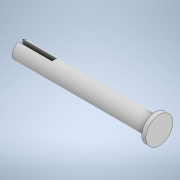
# Autodesk Inventor part: handle insert
Saved by Autodesk Inventor 2020.4 (Build 244396000, 396)
## iProperties
Created: 2023-07-18
Part Number: handle insert
Material: Generic
Document SubType Name: Modeling
Designer: Paul
Density: 1 g/cm^3
Appearance: Default
Author: Paul
Autodesk Inventor part; units mm, degrees
ref_plane "YZ Plane" through (0, 0, 0) normal (1, 0, 0) x (0, 1, 0)
ref_plane "XZ Plane" through (0, 0, 0) normal (0, 1, 0) x (-1, 0, 0)
ref_plane "XY Plane" through (0, 0, 0) normal (0, 0, 1) x (1, 0, 0)
sketch "Sketch1" plane through (0, 0, 0) normal (1, 0, 0) x (0, 1, 0)
  circle A0 centre (0, 0) radius 6.35
  dimension "d0" = 12.7
  constraints: 1 centre point, 1 coincident
  measures "d0" diameter of A0
extrude "Extrusion1" add sketch "Sketch1" along normal mid plane 101.6
sketch "Sketch2" plane through (50.8, 0, 0) normal (1, 0, 0) x (0, 0, -1)
  circle A0 centre (0, 0) radius 10.16
  dimension "d3" = 20.32
  constraints: 1 centre point, 1 coincident
  measures "d3" diameter of A0
extrude "Extrusion2" add sketch "Sketch2" along normal blind 3.175
sketch "Sketch3" plane through (-50.8, 0, 0) normal (-1, 0, 0) x (0, 0, 1)
  line L0 (-1.5875, 3.175) -> (-1.5875, 9.525)
  line L1 (-1.5875, 9.525) -> (1.5875, 9.525)
  line L2 (1.5875, 9.525) -> (1.5875, 3.175)
  line L3 (1.5875, 3.175) -> (-1.5875, 3.175)
  circle A0 centre (0, 0) radius 6.35 projected
  line L4 (-1.5875, 3.175) -> (1.5875, 9.525) construction
  line L5 (-1.5875, 9.525) -> (1.5875, 3.175) construction
  point P0 (0, 6.35)
  dimension "d6" = 6.35
  dimension "d7" = 3.175
  constraints: 12 end point, 2 midpoint, 2 parallel, 1 perpendicular, 1 vertical, 1 vertical alignment, 1 other
  measures "d6" distance of L0.start L0.end
  measures "d7" distance of L0.end L1.end
extrude "Extrusion3" cut sketch "Sketch3" against normal blind 25.4 contours L0 A0 L2 L3 | L0 L1 L2 A0 picked at (-0.1781, 4.2258)
sketch "Sketch4" plane through (-50.8, 3.175, 1.5875) normal (0, 0, -1) x (-1, 0, 0)
  point P0 (-50.8, -3.175)
body "Solid1"
